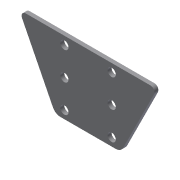
# Autodesk Inventor part: Belt plate top
Saved by Autodesk Inventor 2015 SP1 (Build 190203100, 203)
## iProperties
Created: 2015-01-18
Part Number: Belt plate top
Material: Generic
Document SubType Name: Sheet Metal
Designer: Owner
Density: 1 g/cm^3
Sheet Metal Rule: Default
Appearance: Default
Author: Owner
Autodesk Inventor part; units mm, degrees
ref_plane "YZ Plane" through (0, 0, 0) normal (1, 0, 0) x (0, 1, 0)
ref_plane "XZ Plane" through (0, 0, 0) normal (0, 1, 0) x (-1, 0, 0)
ref_plane "XY Plane" through (0, 0, 0) normal (0, 0, 1) x (1, 0, 0)
sketch "Sketch1" plane through (0, 0, 0) normal (0, 0, 1) x (1, 0, 0)
  line L0 (0, 0) -> (50.8, 0)
  line L1 (-50.8, 101.6) -> (101.6, 101.6)
  line L2 (50.8, 0) -> (78.8, 56)
  line L3 (-28, 56) -> (0, 0)
  line L4 (14.6239, 7) -> (34.6239, 7)
  line L5 (34.6239, 7) -> (34.6239, 2)
  line L6 (34.6239, 2) -> (14.6239, 2)
  line L7 (14.6239, 2) -> (14.6239, 7)
  line L8 (50.8, 0) -> (50.8, 62.4863)
  line L9 (14.6239, 14) -> (34.6239, 14)
  line L10 (34.6239, 14) -> (34.6239, 9)
  line L11 (34.6239, 9) -> (14.6239, 9)
  line L12 (14.6239, 9) -> (14.6239, 14)
  line L13 (14.6239, 21) -> (34.6239, 21)
  line L14 (34.6239, 21) -> (34.6239, 16)
  line L15 (34.6239, 16) -> (14.6239, 16)
  line L16 (14.6239, 16) -> (14.6239, 21)
  line L17 (14.6239, 28) -> (34.6239, 28)
  line L18 (34.6239, 28) -> (34.6239, 23)
  line L19 (34.6239, 23) -> (14.6239, 23)
  line L20 (14.6239, 23) -> (14.6239, 28)
  line L21 (14.6239, 35) -> (34.6239, 35)
  line L22 (34.6239, 35) -> (34.6239, 30)
  line L23 (34.6239, 30) -> (14.6239, 30)
  line L24 (14.6239, 30) -> (14.6239, 35)
  line L25 (14.6239, 42) -> (34.6239, 42)
  line L26 (34.6239, 42) -> (34.6239, 37)
  line L27 (34.6239, 37) -> (14.6239, 37)
  line L28 (14.6239, 37) -> (14.6239, 42)
  circle A0 centre (43.7057, 6.2222) radius 3.1623
  circle A1 centre (43.7057, 28) radius 3.1623
  circle A2 centre (43.7057, 49.7778) radius 3.1623
  line L29 (25.4, 0) -> (25.4, -15.6085)
  circle A3 centre (7.0943, 49.7778) radius 3.1623
  circle A4 centre (7.0943, 6.2222) radius 3.1623
  circle A5 centre (7.0943, 28) radius 3.1623
  line L30 (34.6239, 44) -> (14.6239, 44)
  line L31 (14.6239, 44) -> (14.6239, 49)
  line L32 (34.6239, 49) -> (34.6239, 44)
  line L33 (14.6239, 49) -> (34.6239, 49)
  line L34 (34.6239, 51) -> (14.6239, 51)
  line L35 (14.6239, 51) -> (14.6239, 56)
  line L36 (14.6239, 56) -> (34.6239, 56)
  line L37 (34.6239, 56) -> (34.6239, 51)
  circle A6 centre (-34.29, 91.44) radius 3.1623
  circle A7 centre (85.09, 91.44) radius 3.1623
  line L38 (-28, 56) -> (78.8, 56)
  dimension "d8" = 50.8
  dimension "d9" = 152.4
  dimension "d10" = 101.6
  dimension "d11" = 50.8
  dimension "d12" = 20
  dimension "d13" = 5
  dimension "d14" = 2
  dimension "d15" = 7
  dimension "d16" = 6.3246
  dimension "d17" = 6.3246
  dimension "d18" = 6.3246
  dimension "d19" = 14
  dimension "d20" = 56
  dimension "d21" = 6.2222
  dimension "d22" = 6.2222
  dimension "d23" = 28
  dimension "d24" = 6.3246
  dimension "d25" = 6.3246
  dimension "d26" = 34.29
  dimension "d27" = 34.29
  dimension "d28" = 10.16
  dimension "d29" = 10.16
  measures "d8" distance of L0.start L0.end
  measures "d9" distance of L1.start L1.end
  measures "d10" distance between parallel lines of L1 L0
  measures "d11" horizontal distance of L1.end L0.end
  measures "d12" distance of L5.end L6.end
  measures "d13" distance between parallel lines of L4 L6
  measures "d14" distance between parallel lines of L0 L6
  measures "d15" distance of L4.start L9.start
  measures "d16" diameter of A0
  measures "d17" diameter of A1
  measures "d18" diameter of A2
  measures "d19" distance of L23.end L30.end
  measures "d20" distance between parallel lines of L0 L36
  measures "d21" distance from line of L36 A2.centre
  measures "d22" distance from line of L0 A0.centre
  measures "d23" distance from line of L0 A1.centre
  measures "d24" diameter of A6
  measures "d25" diameter of A7
  measures "d26" horizontal distance of A7.centre L0.end
  measures "d27" horizontal distance of A6.centre L0.start
  measures "d28" vertical distance of A6.centre L1.start
  measures "d29" vertical distance of A7.centre L1.end
extrude "Plate1" add sketch "Sketch1" along normal blind 3.048 contours L3 L38 L35 L34 L37 L8 L0 | L8 L38 L2 | L36 L37 L34 L35 | L4 L5 L6 L7 | L9 L10 L11 L12 | L13 L14 L15 L16 | L17 L18 L19 L20 | L21 L22 L23 L24 | L25 L26 L27 L28 | L30 L31 L33 L32
fillet "Corner Round1" radius 6.35 2 edges at (0, 0, 1.524) (50.8, 0, 1.524)
fillet "Corner Round1" radius 3.175 2 edges at (-28, 56, 1.524) (78.8, 56, 1.524)
equation "\"d17\" = d16"
equation "\"d18\" = d17"
equation "\"d21\" = 0.111111 * d20"
equation "\"d22\" = d21"
equation "\"d23\" = 0.5 * d20"
equation "\"d27\" = d26"
equation "\"d29\" = d28"
equation "\"BendRadius\" = Thickness"
equation "\"BendReliefWidth\" = Thickness"
equation "\"BendReliefDepth\" = 0.5 * Thickness"
equation "\"CornerReliefSize\" = 4 * Thickness"
equation "\"MinimumRemnant\" = 2 * Thickness"
equation "\"TransitionRadius\" = BendRadius"
equation "\"JacobiRadiusSize\" = BendRadius"
equation "\"GapSize\" = Thickness"
equation "\"d32\" = BendRadius"
equation "\"Thickness\" = 3.048"
body "Solid1"
